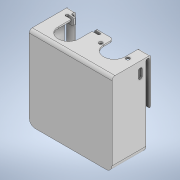
# Autodesk Inventor part: UniversalMount_v1
Saved by Autodesk Inventor 2021 (Build 250183000, 183)
## iProperties
Created: 2021-02-23
Part Number: UniversalMount_v1
Material: Generic
Document SubType Name: Modeling
Designer: allen
Density: 1 g/cm^3
Appearance: Default
Author: allen
Autodesk Inventor part; units mm, degrees
ref_plane "YZ Plane" through (0, 0, 0) normal (1, 0, 0) x (0, 1, 0)
ref_plane "XZ Plane" through (0, 0, 0) normal (0, 1, 0) x (-1, 0, 0)
ref_plane "XY Plane" through (0, 0, 0) normal (0, 0, 1) x (1, 0, 0)
sketch "Sketch1" plane through (0, 0, 0) normal (0, 0, 1) x (1, 0, 0)
  line L0 (-55, -55) -> (55, -55)
  line L1 (55, -55) -> (55, 55)
  line L2 (55, 55) -> (-55, 55)
  line L3 (-55, 55) -> (-55, -55)
  line L4 (-55, -55) -> (55, 55) construction
  line L5 (55, -55) -> (-55, 55) construction
  point P0 (0, 0)
  dimension "d0" = 110
  dimension "d1" = 110
  constraints: 12 end point, 2 midpoint, 2 parallel, 1 horizontal, 1 perpendicular
  measures "d0" distance of L1.end L2.end
  measures "d1" distance of L2.end L0.start
extrude "Extrusion1" add sketch "Sketch1" along normal blind 45
sketch "Sketch8" plane through (-55, 55, 0) normal (0, 1, 0) x (1, 0, 0)
  arc A0 (16.125, -22.8) -> (43.875, -22.8) centre (30, -22.8) ccw
  line L0 (110, 0) -> (0, 0) projected
  line L1 (43.875, -22.8) -> (43.875, 0)
  line L2 (16.125, -22.8) -> (16.125, 0)
  line L3 (43.875, 0) -> (16.125, 0)
  line L4 (0, 0) -> (0, -45) projected
  point P0 (55, 0)
  dimension "d22" = 22.8
  dimension "d23" = 30
  dimension "d24" = 22.8
  dimension "d25" = 22.8
  dimension "d33" = 13.875
  constraints: 6 end point, 2 perpendicular, 2 point on circle, 2 point on line, 1 centre point, 1 collinear
  measures "d22" distance from line of L0 A0.centre
  measures "d23" distance from line of L4 A0.centre
  measures "d24" distance of L2.start L2.end
  measures "d25" distance of L1.start L1.end
  measures "d33" radius of A0
sketch "Sketch9" plane through (0, 0, 0) normal (0, 0, -1) x (-1, 0, 0)
  line L0 (-53, -53) -> (53, -53)
  line L1 (53, -53) -> (53, 53)
  line L2 (53, 53) -> (-53, 53)
  line L3 (-53, 53) -> (-53, -53)
  line L4 (-53, -53) -> (53, 53) construction
  line L5 (53, -53) -> (-53, 53) construction
  line L6 (55, 55) -> (55, -55) projected
  line L7 (-55, 55) -> (55, 55) projected
  point P0 (0, 0)
  dimension "d27" = 2
  dimension "d28" = 2
  constraints: 12 end point, 2 midpoint, 2 parallel, 1 horizontal, 1 perpendicular
  measures "d27" distance between parallel lines of L6 L1
  measures "d28" distance between parallel lines of L2 L7
extrude "Extrusion5" cut sketch "Sketch9" against normal blind 43
extrude "Extrusion6" cut sketch "Sketch8" against normal blind 38
sketch "Sketch10" plane through (0, 0, 0) normal (0, 0, -1) x (-1, 0, 0)
  line L0 (-55, 55) -> (11.125, 55) projected
  line L1 (11.125, 55) -> (-2.875, 55)
  line L2 (-2.875, 55) -> (-2.875, 45)
  line L3 (-2.875, 45) -> (11.125, 45)
  line L4 (11.125, 45) -> (11.125, 55)
  line L5 (38.875, 55) -> (38.875, 53) projected
  line L6 (38.875, 55) -> (54.875, 55)
  line L7 (54.875, 55) -> (54.875, 45)
  line L8 (54.875, 45) -> (38.875, 45)
  line L9 (38.875, 45) -> (38.875, 55)
  circle A0 centre (6.875, 50.5) radius 1.4
  circle A1 centre (43.375, 50.5) radius 1.4
  line L10 (-53, 53) -> (11.125, 53) projected
  line L11 (38.875, 53) -> (53, 53) projected
  point P0 (0, 0)
  dimension "d34" = 10
  dimension "d35" = 14
  dimension "d36" = 2.8
  dimension "d39" = 2.8
  dimension "d42" = 36.5
  dimension "d43" = 4.25
  dimension "d44" = 16
  dimension "d47" = 2.5
  dimension "d48" = 2.5
  constraints: 16 end point, 5 parallel, 2 centre point, 2 horizontal, 2 perpendicular
  measures "d34" distance of L1.end L2.end
  measures "d35" distance of L2.end L3.end
  measures "d36" diameter of A0
  measures "d39" diameter of A1
  measures "d42" distance between centres of A0 A1
  measures "d43" distance from line of L4 A0.centre
  measures "d44" distance of L7.end L8.end
  measures "d47" distance from line of A0.centre L10
  measures "d48" distance from line of L11 A1.centre
extrude "Extrusion7" add sketch "Sketch10" against normal blind 2
sketch "Sketch12" plane through (0, 0, 2) normal (0, 0, 1) x (1, 0, 0)
  line L0 (-2.125, 14.72) -> (-47.875, 14.72)
  line L1 (-47.875, 14.72) -> (-47.875, 55.3239)
  line L2 (-47.875, 55.3239) -> (-2.125, 55.3239)
  line L3 (-2.125, 55.3239) -> (-2.125, 14.72)
  line L4 (-38.875, 55) -> (-38.875, 45) projected
  line L5 (-11.125, 45) -> (-11.125, 55) projected
  point P0 (0, 0)
  dimension "d54" = 9
  dimension "d55" = 9
  constraints: 8 end point, 2 parallel, 1 horizontal, 1 perpendicular
  measures "d54" distance between parallel lines of L4 L1
  measures "d55" distance between parallel lines of L5 L3
extrude "Extrusion9" cut sketch "Sketch12" along normal blind 3.3
fillet "Fillet4" radius 1.5 10 edges at (-2.125, 54, 5.3) (-2.125, 54, 2) (-47.875, 54, 2) (-47.875, 54, 5.3) (-38.875, 54, 5.3) (-11.125, 54, 5.3) (-11.125, 55, 1) (-38.875, 55, 1) (-38.875, 45, 1) (-11.125, 45, 1)
sketch "Sketch13" plane through (-25, 55, 22.8) normal (0, 1, 0) x (1, 0, 0)
  arc A0 (37, 9.8) -> (65, 9.8) centre (51, 9.8) ccw
  line L0 (65, 9.8) -> (65, 22.8)
  line L1 (-28, 22.8) -> (78, 22.8) projected
  line L2 (37, 9.8) -> (37, 22.8)
  line L3 (100, -21.8) -> (100, 18.2) projected
  line L4 (51, 9.8) -> (51, -12.8982) construction
  circle A1 centre (69, 9.8) radius 2.5
  circle A2 centre (33, 9.8) radius 2.5
  point P0 (25, 22.8)
  point P1 (-26, 18.2)
  point P2 (96, 18.2)
  dimension "d61" = 13
  dimension "d62" = 13
  dimension "d63" = 14
  dimension "d64" = 35
  dimension "d65" = 18
  dimension "d66" = 5
  dimension "d67" = 13
  constraints: 6 end point, 3 centre point, 2 point on circle, 2 vertical, 1 parallel, 1 symmetric about line, 1 tangent, 4 other
  measures "d61" distance of L2.start L2.end
  measures "d62" distance of L0.start L0.end
  measures "d63" radius of A0
  measures "d64" distance between parallel lines of L3 L0
  measures "d65" distance from line of L4 A1.centre
  measures "d66" diameter of A1
extrude "Extrusion10" cut sketch "Sketch13" against normal blind 2
sketch "Sketch16" plane through (-25, 53, 22.8) normal (0, -1, 0) x (1, 0, 0)
  line L0 (27.9547, -18.2) -> (26.4675, -18.2) projected
  line L1 (27.9547, -18.2) -> (23.375, -18.2)
  line L2 (23.375, -18.2) -> (23.375, -10.2)
  line L3 (23.375, -10.2) -> (27.9547, -10.2)
  line L4 (27.9547, -10.2) -> (27.9547, -18.2)
  line L5 (22.875, -19) -> (22.875, -19.3) projected
  point P0 (25, -22.8)
  point P1 (26.4675, -18.2)
  dimension "d83" = 8
  dimension "d84" = 0.5
  constraints: 8 end point, 2 parallel, 1 horizontal, 1 perpendicular
  measures "d83" distance of L1.end L2.end
  measures "d84" distance between parallel lines of L5 L2
extrude "Extrusion13" add sketch "Sketch16" along normal blind 5
fillet "Fillet8" radius 2 2 edges at (0.6648, 48, 12.6) (0.6648, 53, 12.6)
sketch "Sketch18" plane through (-55, -55, 0) normal (-1, 0, 0) x (0, 0, 1)
  line L0 (0, 108) -> (0, 110) projected
  line L1 (0, 110) -> (-6.5, 110)
  line L2 (-6.5, 110) -> (-6.5, 50)
  line L3 (-6.5, 50) -> (-4.5, 50)
  line L4 (0, 100) -> (0, 2) projected
  line L5 (-4.5, 50) -> (-4.5, 108)
  line L6 (0, 108.5) -> (0, 101.5) projected
  line L7 (-4.5, 108) -> (0, 108)
  point P0 (0, 55)
  dimension "d88" = 4.5
  dimension "d89" = 60
  dimension "d90" = 6.5
  dimension "d91" = 2
  constraints: 10 end point, 3 perpendicular, 1 horizontal, 1 parallel, 1 point on line
  measures "d88" distance of L5.end L7.end
  measures "d89" distance of L1.end L2.end
  measures "d90" distance of L0.end L1.end
  measures "d91" distance between parallel lines of L1 L7
extrude "Extrusion14" add sketch "Sketch18" against normal blind 10
sketch "Sketch19" plane through (55, -55, 0) normal (1, 0, 0) x (0, 0, -1)
  line L0 (0, 110) -> (-2, 110) projected
  line L1 (6.5, 110) -> (0, 110) projected
  line L2 (0, 110) -> (6.5, 110)
  line L3 (6.5, 50) -> (6.5, 110) projected
  line L4 (6.5, 110) -> (6.5, 50)
  line L5 (4.5, 50) -> (6.5, 50) projected
  line L6 (6.5, 50) -> (4.5, 50)
  line L7 (0, 108) -> (4.5, 108) projected
  line L8 (4.5, 50) -> (4.5, 108)
  line L9 (4.5, 108) -> (0, 108)
  line L10 (0, 108) -> (0, 110)
  point P0 (0, 55)
  constraints: 12 end point, 4 perpendicular, 2 collinear
extrude "Extrusion15" add sketch "Sketch19" against normal blind 15
fillet "Fillet9" radius 2 9 edges at (-50, 55, -6.5) (-50, 53, -4.5) (-50, -5, -6.5) (-50, 53, 0) (47.5, 53, -4.5) (47.5, 55, -6.5) (47.5, -5, -6.5) (54, 53, 0) (-45, 54, 0)
fillet "Fillet10" radius 8 4 edges at (55, -55, 22.5) (53, -53, 21.5) (-55, -55, 22.5) (-53, -53, 21.5)
sketch "Sketch20" plane through (53, 53, -2) normal (-1, 0, 0) x (0, 0, 1)
  line L0 (12, -6) -> (7, -6)
  line L1 (7, -6) -> (7, -19)
  line L2 (7, -19) -> (12, -19)
  line L3 (12, -19) -> (12, -6)
  line L4 (-2.5, 2) -> (47, 2) projected
  line L5 (2, -98) -> (2, -2) projected
  point P0 (2, -53)
  dimension "d98" = 13
  dimension "d99" = 5
  dimension "d100" = 8
  dimension "d101" = 5
  constraints: 8 end point, 2 parallel, 1 horizontal, 1 perpendicular
  measures "d98" distance of L0.end L1.end
  measures "d99" distance of L1.end L2.end
  measures "d100" distance between parallel lines of L4 L0
  measures "d101" distance between parallel lines of L5 L1
extrude "Extrusion16" cut sketch "Sketch20" against normal blind 10
fillet "Fillet11" radius 2 4 edges at (54, 47, 5) (54, 47, 10) (54, 34, 10) (54, 34, 5)
sketch "Sketch21" plane through (-45, -53, 0) normal (0, 1, 0) x (1, 0, 0)
  circle A0 centre (84, -35) radius 4
  line L0 (-2, -45) -> (92, -45) projected
  line L1 (100, 0) -> (100, -45) projected
  point P0 (45, 0)
  dimension "d105" = 8
  dimension "d106" = 10
  dimension "d107" = 16
  constraints: 1 centre point
  measures "d105" diameter of A0
  measures "d106" distance from line of L0 A0.centre
  measures "d107" distance from line of L1 A0.centre
extrude "Extrusion17" cut sketch "Sketch21" against normal blind 10
fillet "Fillet12" radius 4 2 edges at (0, 55, 45) (0, 53, 43)
fillet "Fillet13" radius 4 3 edges at (12, 54, 0) (2.9547, 53, 9.6) (2.875, 45, 1)
body "Solid1"
